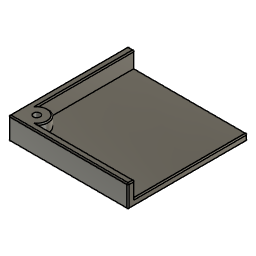
pcb_side_hole_drill_helper (Autodesk Fusion 360 design; units mm, degrees)
part number: 2025-06-30-21-36-17-882
Autodesk Fusion 360 part; units mm, degrees
note: some values were not read from the file. Set by a fixed rule: which sketch regions a step uses.
sketch "Sketch1" plane through (0, 0, 0) normal (0, 0, 1) x (1, 0, 0)
  line L0 (0, 0) -> (50, 0)
  line L1 (50, 0) -> (50, 50)
  line L2 (50, 50) -> (0, 50)
  line L3 (0, 50) -> (0, 0)
  dimension "d1" = 50
  dimension "d2" = 50
  constraint horizontal L0
  constraint vertical L1
  constraint horizontal L2
  constraint vertical L3
  constraint coincident L0.start L3.end
  measures "d1" distance of L0.start L0.end
  measures "d2" distance of L0.start L2.end
extrude "Extrude1" add sketch "Sketch1" along normal blind 3
sketch "Sketch2" plane through (0, 0, 0) normal (0, 0, 1) x (1, 0, 0)
  line L0 (50, 50) -> (0, 50)
  line L1 (50, 0) -> (50, 50)
  line L2 (0, 0) -> (50, 0)
  line L3 (0, 50) -> (0, 0)
  line L4 (-3, 50) -> (-3, -3)
  line L5 (-3, -3) -> (50, -3)
  line L6 (-3, 50) -> (0, 50)
  line L7 (50, 0) -> (50, -3)
  dimension "d8" = 3
  constraint coincident L0.end L3.start
  constraint perpendicular L3 L6
  constraint coincident L1.start L2.end
  constraint perpendicular L5 L7
extrude "Extrude2" add sketch "Sketch2" along normal blind 10 contours L2 L3 L4 L5 L6 L7
ref_plane "WorkPlane1" through (25, 25, 5.5) normal (0, 0, 1) x (1, 0, 0)
sketch "Sketch4" plane through (0, 0, 5.5) normal (0, 0, 1) x (1, 0, 0)
  circle A0 centre (3.25, 3.25) radius 5
  line L0 (0, 0) -> (0, 50)
  line L1 (50, 0) -> (0, 0)
  dimension "d15" = 3.25
  dimension "d16" = 3.25
  dimension "d25" = 10
  measures "d15" distance of A0.centre L0
  measures "d16" distance of A0.centre L1
  measures "d25" diameter of A0
extrude "Extrude3" add sketch "Sketch4" along normal blind 4.5 contours A0 L0 L1 picked at (4.5229, 4.5125)
sketch "Sketch5" plane through (0, 0, 10) normal (0, 0, 1) x (-1, 0, 0)
  line L0 (3, -50) -> (3, 3)
  line L1 (3, 3) -> (-50, 3)
  line L2 (-50, 3) -> (-50, 0)
  line L3 (-50, 0) -> (-7.0497, 0)
  arc A0 (-7.0497, 0) -> (0, -7.0497) centre (-3.25, -3.25) ccw
  line L4 (0, -7.0497) -> (0, -50)
  line L5 (0, -50) -> (3, -50)
hole "Hole2" at (3.25, 3.25, 10) direction (0, 0, -1) diameter 3 end up to surface (10 mm away)
fillet "Fillet1" radius 0.5 12 edges at (23.5, -3, 0) (50, -3, 5) (23.5, -3, 10) (-3, -3, 5) (-3, 23.5, 0) (-3, 23.5, 10) (23.5, 50, 0) (50, 23.5, 0) (-1.5, 50, 10) (-3, 50, 5) (50, -1.5, 10) (50, 50, 1.5)
fillet "Fillet2" radius 0.5 10 edges at (50, 0, 6.25) (49.8536, 0, 9.8536) (28.2748, 0, 10) (0, 28.2748, 10) (0, 49.8536, 9.8536) (0, 50, 6.25) (50, 24.75, 3) (49.8536, 49.8536, 3) (24.75, 50, 3) (6.7855, 6.7855, 10)
equation "d16 = d15"
equation "d17 = 7 mm - 2.5 mm"
